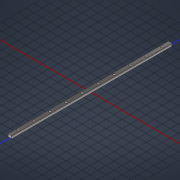
# Autodesk Inventor part: Linear-Rail MGN9h (400mm)
Saved by Autodesk Inventor 2022.2 (Build 262287010, 287A)
## iProperties
Created: 2022-03-13
Part Number: Linear-Rail MGN9h (400mm)
Material: Stahl, hochfest, niedrig legiert
Document SubType Name: Modeling
Designer: sleib
Density: 7.85 g/cm^3
Appearance: Stahl - poliert
Author: sleib
Autodesk Inventor part; units mm, degrees
ref_plane "YZ Plane" through (0, 0, 0) normal (1, 0, 0) x (0, 1, 0)
ref_plane "XZ Plane" through (0, 0, 0) normal (0, 1, 0) x (-1, 0, 0)
ref_plane "XY Plane" through (0, 0, 0) normal (0, 0, 1) x (1, 0, 0)
sketch "Skizze1" plane through (0, 0, 0) normal (0, 0, 1) x (1, 0, 0)
  arc A0 (-3.6501, 1.7625) -> (-4.5, 2.445) centre (-4.6, 1.45) ccw
  line L0 (-3.6501, 1.7625) -> (-3.1501, 1.7625)
  line L1 (-3.1501, 1.7625) -> (-3.1501, 1.2625)
  line L2 (-3.1501, 1.2625) -> (-3.6177, 1.2625)
  arc A1 (-4.5, 0.455) -> (-3.6177, 1.2625) centre (-4.6, 1.45) ccw
  line L3 (-4.5, 0.455) -> (-4.5, -3.05)
  line L4 (-4.5, -3.05) -> (-4.3, -3.25)
  line L5 (-4.3, -3.25) -> (4.3, -3.25)
  line L6 (4.3, -3.25) -> (4.5, -3.05)
  line L7 (4.5, -3.05) -> (4.5, 0.455)
  arc A2 (3.6177, 1.2625) -> (4.5, 0.455) centre (4.6, 1.45) ccw
  line L8 (3.6177, 1.2625) -> (3.1501, 1.2625)
  line L9 (3.1501, 1.2625) -> (3.1501, 1.7625)
  line L10 (3.1501, 1.7625) -> (3.6501, 1.7625)
  arc A3 (4.5, 2.445) -> (3.6501, 1.7625) centre (4.6, 1.45) ccw
  line L11 (4.5, 2.445) -> (4.5, 3.05)
  line L12 (4.5, 3.05) -> (4.3, 3.25)
  line L13 (4.3, 3.25) -> (-4.3, 3.25)
  line L14 (-4.3, 3.25) -> (-4.5, 3.05)
  line L15 (-4.5, 3.05) -> (-4.5, 2.445)
  circle A4 centre (-4.6, 1.45) radius 1 construction
  circle A5 centre (4.6, 1.45) radius 1 construction
  line L16 (0, -4.55) -> (0, 4.55) construction
  point P0 (0, 0)
  point P1 (0, 0)
  point P2 (0, 3.25)
  point P3 (0, -3.25)
  dimension "d0" = 9
  dimension "d1" = 6.5
  dimension "d2" = 4.7
  dimension "d4" = 2
  dimension "d5" = 6.3002
  dimension "d6" = 0.5
  dimension "d7" = 0.4499
  dimension "d8" = 3.25
  dimension "d12" = 0.2
  dimension "d13" = 0.2
  dimension "d18" = 1.4875
  constraints: 32 end point, 8 point on circle, 6 centre point, 4 coincident, 4 collinear, 4 concentric, 4 horizontal alignment, 2 midpoint, 2 perpendicular, 2 point on line, 2 vertical alignment, 1 equal radius, 1 horizontal, 1 symmetric about line, 2 other
  measures "d0" distance between parallel lines of L7 L3
  measures "d1" distance between parallel lines of L5 L13
  measures "d2" distance from line of L5 A1.centre
  measures "d4" diameter of A4
  measures "d5" distance between parallel lines of L1 L9
  measures "d6" distance between parallel lines of L2 L0
  measures "d7" distance edge to line of A4 L1
  measures "d8" distance from line of L5 point (0, 0)
  measures "d12" horizontal distance of L5.start L4.start
  measures "d13" horizontal distance of L5.start L4.start
  measures "d18" distance between parallel lines of L13 L0
extrude "Extrusion1" add sketch "Skizze1" along normal mid plane 400
sketch "Skizze2" plane through (-4.3, 3.25, 200) normal (0, 1, 0) x (1, 0, 0)
  line L0 (0, 400) -> (0, 0) projected
  line L1 (8.6, 0) -> (0, 0) projected
  line L2 (8.6, 400) -> (8.6, 0) projected
  line L3 (0, 400) -> (8.6, 400) projected
  line L4 (8.6, 0) -> (0, 0) projected
  line L5 (4.3, 0) -> (4.3, 400) construction
  line L6 (0, 400) -> (8.6, 400) projected
  line L7 (0, 400) -> (0, 0) projected
  line L8 (0, 200) -> (8.6, 200) construction
  line L9 (8.6, 400) -> (8.6, 0) projected
  point P0 (4.3, 20)
  point P1 (4.3, 60)
  point P2 (4.3, 100)
  point P3 (4.3, 140)
  point P4 (4.3, 180)
  point P5 (4.3, 220)
  point P6 (4.3, 260)
  point P7 (4.3, 300)
  point P8 (4.3, 340)
  point P9 (4.3, 380)
  dimension "d23" = 40
  dimension "d28" = 20
  constraints: 4 end point, 4 midpoint, 1 point on line, 1 vertical, 9 other
  measures "d23" distance of point (4.3, 20) point (4.3, 60)
  measures "d28" distance from line of point (4.3, 20) L1
hole "Bohrung1" at (0, 3.25, 180) at (0, 3.25, 140) at (0, 3.25, 100) at (0, 3.25, 60) at (0, 3.25, 20) at (0, 3.25, -20) at (0, 3.25, -60) at (0, 3.25, -100) at (0, 3.25, -140) at (0, 3.25, -180) direction (0, -1, 0) diameter 3.4 end through all counterbore diameter 6 counterbore depth 3.4 clearance for "Inbusschraube DIN EN ISO 4762" size "M3" standard "DIN"
chamfer "Fase1" distance 0.25 angle 45 10 edges at (0, 3.25, 177) (0, 3.25, 137) (0, 3.25, 97) (0, 3.25, 57) (0, 3.25, 17) (0, 3.25, -23) (0, 3.25, -63) (0, 3.25, -103) (0, 3.25, -143) (0, 3.25, -183)
